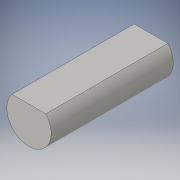
# Autodesk Inventor part: Motor Shaft
Saved by Autodesk Inventor 2016 SP1 (Build 200210100, 210)
## iProperties
Created: 2016-04-13
Part Number: Motor Shaft
Material: Generic
Document SubType Name: Modeling
Designer: schiu30
Density: 1 g/cm^3
Appearance: Default
Author: schiu30
Autodesk Inventor part; units mm, degrees
ref_plane "YZ Plane" through (0, 0, 0) normal (1, 0, 0) x (0, 1, 0)
ref_plane "XZ Plane" through (0, 0, 0) normal (0, 1, 0) x (-1, 0, 0)
ref_plane "XY Plane" through (0, 0, 0) normal (0, 0, 1) x (1, 0, 0)
sketch "Sketch1" plane through (0, 0, 0) normal (0, 0, 1) x (1, 0, 0)
  arc A0 (-1.5199, 1.3) -> (1.5199, 1.3) centre (0, 0) ccw
  line L0 (-1.5199, 1.3) -> (1.5199, 1.3)
  dimension "d0" = 4
  dimension "d1" = 3.3
  constraints: 2 end point, 2 point on circle, 1 centre point, 1 coincident, 1 horizontal
  measures "d0" diameter of A0
extrude "Extrusion1" add sketch "Sketch1" along normal blind 11
body "Solid1"
